Autodesk Fusion 360 part; units mm, degrees
(part 3 of 3)
sketch "Skizze23" plane through (0, 0, 15) normal (0, 0, 1) x (-1, 0, 0)
  circle A0 centre (-5.0127, -12.7944) radius 1.5
  circle A1 centre (-7.0127, 10.2056) radius 1.5
  circle A2 centre (20.7786, -30.2009) radius 1.5
  circle A3 centre (-14.804, -30.2009) radius 1.5
  circle A4 centre (12.9873, -19.7944) radius 1.5
  circle A5 centre (12.9873, 10.2056) radius 1.5
  circle A6 centre (-5.0127, 3.2056) radius 1.5
  circle A7 centre (10.9873, -12.7944) radius 1.5
  circle A8 centre (-16.9122, 11.6198) radius 1.5
  circle A9 centre (10.9873, -60.7944) radius 1.5
  circle A10 centre (-5.0127, -60.7944) radius 1.5
  circle A11 centre (-7.0127, -19.7944) radius 1.5
  circle A12 centre (22.8868, 11.6198) radius 1.5
  circle A13 centre (10.9873, 3.2056) radius 1.5
  circle A14 centre (12.9873, -49.2944) radius 1
  arc A15 (10.4462, -52.3625) -> (9.4415, -47.3835) centre (3.5497, -51.1632) ccw
  line L0 (10.4462, -52.3625) -> (9.904, -55.4797)
  arc A16 (5.9632, -58.7944) -> (9.904, -55.4797) centre (5.9632, -54.7944) ccw
  line L1 (5.9632, -58.7944) -> (0.0113, -58.7944)
  arc A17 (-3.9295, -55.4797) -> (0.0113, -58.7944) centre (0.0113, -54.7944) ccw
  line L2 (-3.9295, -55.4797) -> (-4.4716, -52.3625)
  arc A18 (-3.467, -47.3835) -> (-4.4716, -52.3625) centre (2.4249, -51.1632) ccw
  line L3 (-3.467, -47.3835) -> (1.9547, -38.932)
  arc A19 (2.7964, -38.4719) -> (1.9547, -38.932) centre (2.7964, -39.4719) ccw
  line L4 (2.7964, -38.4719) -> (3.1781, -38.4719)
  arc A20 (4.0198, -38.932) -> (3.1781, -38.4719) centre (3.1781, -39.4719) ccw
  line L5 (4.0198, -38.932) -> (9.4415, -47.3835)
  arc A21 (-4.7211, -31.3597) -> (-5.0127, -32.7585) centre (-1.5127, -32.7585) ccw
  arc A22 (-4.7211, -31.3597) -> (-4.5127, -30.3606) centre (-7.0127, -30.3606) ccw
  line L6 (-4.5127, -30.3606) -> (-4.5127, -28.821)
  arc A23 (-2.6684, -28.2852) -> (-4.5127, -28.821) centre (-3.5127, -28.821) ccw
  line L7 (-2.6684, -28.2852) -> (-0.2775, -32.0531)
  arc A24 (0.0338, -33.1247) -> (-0.2775, -32.0531) centre (-1.9662, -33.1247) ccw
  line L8 (0.0338, -33.1247) -> (0.0338, -35.784)
  arc A25 (-0.2829, -36.8639) -> (0.0338, -35.784) centre (-1.9662, -35.784) ccw
  line L9 (-0.2829, -36.8639) -> (-3.171, -41.3661)
  arc A26 (-5.0127, -40.8261) -> (-3.171, -41.3661) centre (-4.0127, -40.8261) ccw
  line L10 (-5.0127, -40.8261) -> (-5.0127, -32.7585)
  arc A27 (3.1526, -30.4719) -> (3.997, -30.0077) centre (3.1526, -29.4719) ccw
  line L11 (3.1526, -30.4719) -> (2.8219, -30.4719)
  arc A28 (1.9776, -30.0077) -> (2.8219, -30.4719) centre (2.8219, -29.4719) ccw
  line L12 (1.9776, -30.0077) -> (-0.6732, -25.8302)
  arc A29 (0.1711, -24.2944) -> (-0.6732, -25.8302) centre (0.1711, -25.2944) ccw
  line L13 (0.1711, -24.2944) -> (5.8034, -24.2944)
  arc A30 (6.6478, -25.8302) -> (5.8034, -24.2944) centre (5.8034, -25.2944) ccw
  line L14 (6.6478, -25.8302) -> (3.997, -30.0077)
  line L15 (7.9873, 8.7056) -> (-2.0127, 8.7056)
  arc A31 (-2.0127, 11.7056) -> (-2.0127, 8.7056) centre (-2.0127, 10.2056) ccw
  line L16 (-2.0127, 11.7056) -> (7.9873, 11.7056)
  arc A32 (7.9873, 8.7056) -> (7.9873, 11.7056) centre (7.9873, 10.2056) ccw
  line L17 (7.9873, -21.2944) -> (-2.0127, -21.2944)
  arc A33 (-2.0127, -18.2944) -> (-2.0127, -21.2944) centre (-2.0127, -19.7944) ccw
  line L18 (-2.0127, -18.2944) -> (7.9873, -18.2944)
  arc A34 (7.9873, -21.2944) -> (7.9873, -18.2944) centre (7.9873, -19.7944) ccw
  circle A35 centre (-7.0127, -49.2944) radius 1
  line L19 (9.4873, -1.2944) -> (9.4873, -8.2944)
  arc A36 (6.4873, -11.2944) -> (9.4873, -8.2944) centre (6.4873, -8.2944) ccw
  line L20 (6.4873, -11.2944) -> (-0.5127, -11.2944)
  arc A37 (-3.5127, -8.2944) -> (-0.5127, -11.2944) centre (-0.5127, -8.2944) ccw
  line L21 (-3.5127, -8.2944) -> (-3.5127, -1.2944)
  arc A38 (-0.5127, 1.7056) -> (-3.5127, -1.2944) centre (-0.5127, -1.2944) ccw
  line L22 (-0.5127, 1.7056) -> (6.4873, 1.7056)
  arc A39 (9.4873, -1.2944) -> (6.4873, 1.7056) centre (6.4873, -1.2944) ccw
  arc A40 (10.4873, -28.821) -> (8.6429, -28.2852) centre (9.4873, -28.821) ccw
  line L23 (10.4873, -28.821) -> (10.4873, -30.3606)
  arc A41 (10.4873, -30.3606) -> (10.6956, -31.3597) centre (12.9873, -30.3606) ccw
  arc A42 (10.9873, -32.7585) -> (10.6956, -31.3597) centre (7.4873, -32.7585) ccw
  line L24 (10.9873, -32.7585) -> (10.9873, -40.8261)
  arc A43 (9.1456, -41.3661) -> (10.9873, -40.8261) centre (9.9873, -40.8261) ccw
  line L25 (9.1456, -41.3661) -> (6.2574, -36.8639)
  arc A44 (5.9408, -35.784) -> (6.2574, -36.8639) centre (7.9408, -35.784) ccw
  line L26 (5.9408, -35.784) -> (5.9408, -33.1247)
  arc A45 (6.2521, -32.0531) -> (5.9408, -33.1247) centre (7.9408, -33.1247) ccw
  line L27 (6.2521, -32.0531) -> (8.6429, -28.2852)
  circle A46 centre (-7.0127, -29.2944) radius 1
  circle A47 centre (12.9873, -29.2944) radius 1
  arc A48 (14.4873, -45.5527) -> (15.1539, -48.0472) centre (19.4873, -45.5527) ccw
  line L28 (14.4873, -45.5527) -> (14.4873, -33.6896)
  arc A49 (17.1075, -32.6921) -> (14.4873, -33.6896) centre (15.9873, -33.6896) ccw
  line L29 (17.1075, -32.6921) -> (17.4938, -33.1258)
  arc A50 (17.4938, -33.1258) -> (24.5102, -27.8727) centre (20.7786, -30.2009) ccw
  line L30 (24.5102, -27.8727) -> (18.3167, -17.946)
  arc A51 (16.8008, -12.6526) -> (18.3167, -17.946) centre (26.8008, -12.6526) ccw
  line L31 (16.8008, -12.6526) -> (16.8008, 1.4922)
  arc A52 (20.6559, 6.3594) -> (16.8008, 1.4922) centre (21.8008, 1.4922) ccw
  line L32 (20.6559, 6.3594) -> (23.9423, 7.1324)
  arc A53 (23.9423, 7.1324) -> (22.6436, 16.2233) centre (22.8868, 11.6198) ccw
  line L33 (22.6436, 16.2233) -> (5.6243, 15.3244)
  arc A54 (0.3502, 15.3244) -> (5.6243, 15.3244) centre (2.9873, 65.2548) ccw
  line L34 (0.3502, 15.3244) -> (-16.6691, 16.2233)
  arc A55 (-16.6691, 16.2233) -> (-17.9678, 7.1324) centre (-16.9122, 11.6198) ccw
  line L35 (-17.9678, 7.1324) -> (-14.6814, 6.3594)
  arc A56 (-10.8263, 1.4922) -> (-14.6814, 6.3594) centre (-15.8263, 1.4922) ccw
  line L36 (-10.8263, 1.4922) -> (-10.8263, -12.6526)
  arc A57 (-12.3422, -17.946) -> (-10.8263, -12.6526) centre (-20.8263, -12.6526) ccw
  line L37 (-12.3422, -17.946) -> (-18.5356, -27.8727)
  arc A58 (-18.5356, -27.8727) -> (-11.5192, -33.1258) centre (-14.804, -30.2009) ccw
  line L38 (-11.5192, -33.1258) -> (-11.133, -32.6921)
  arc A59 (-8.5127, -33.6896) -> (-11.133, -32.6921) centre (-10.0127, -33.6896) ccw
  line L39 (-8.5127, -33.6896) -> (-8.5127, -45.5527)
  arc A60 (-9.1794, -48.0472) -> (-8.5127, -45.5527) centre (-13.5127, -45.5527) ccw
  arc A61 (-9.1794, -48.0472) -> (-8.9906, -50.8235) centre (-7.0127, -49.2944) ccw
  arc A62 (-8.0346, -52.946) -> (-8.9906, -50.8235) centre (-12.9463, -53.8816) ccw
  line L40 (-8.0346, -52.946) -> (-7.5111, -55.6946)
  arc A63 (-8.0639, -59.0797) -> (-7.5111, -55.6946) centre (-12.4228, -56.6301) ccw
  arc A64 (-8.0639, -59.0797) -> (-3.0273, -63.6767) centre (-5.0127, -60.7944) ccw
  arc A65 (-0.1909, -62.7944) -> (-3.0273, -63.6767) centre (-0.1909, -67.7944) ccw
  line L41 (-0.1909, -62.7944) -> (6.1654, -62.7944)
  arc A66 (9.0018, -63.6767) -> (6.1654, -62.7944) centre (6.1654, -67.7944) ccw
  arc A67 (9.0018, -63.6767) -> (14.0385, -59.0797) centre (10.9873, -60.7944) ccw
  arc A68 (13.4856, -55.6946) -> (14.0385, -59.0797) centre (18.3973, -56.6301) ccw
  line L42 (13.4856, -55.6946) -> (14.0092, -52.946)
  arc A69 (14.9651, -50.8235) -> (14.0092, -52.946) centre (18.9209, -53.8816) ccw
  arc A70 (14.9651, -50.8235) -> (15.1539, -48.0472) centre (12.9873, -49.2944) ccw
sketch "Skizze24" plane through (0, 0, 9) normal (0, 0, 1) x (-1, 0, 0)
  arc A0 (14.9683, -29.0197) -> (16.1868, -31.658) centre (19.9209, -28.333) ccw
  line L0 (16.1868, -31.658) -> (17.4938, -33.1258)
  arc A1 (17.4938, -33.1258) -> (24.5102, -27.8727) centre (20.7786, -30.2009) ccw
  line L1 (24.5102, -27.8727) -> (18.3167, -17.946)
  arc A2 (16.8008, -12.6526) -> (18.3167, -17.946) centre (26.8008, -12.6526) ccw
  line L2 (16.8008, -12.6526) -> (16.8008, 1.4922)
  arc A3 (18.2009, 4.9622) -> (16.8008, 1.4922) centre (21.8008, 1.4922) ccw
  arc A4 (19.0475, 5.6658) -> (18.2009, 4.9622) centre (28.2059, -6.2137) ccw
  arc A5 (20.6559, 6.3594) -> (19.0475, 5.6658) centre (21.8008, 1.4922) ccw
  line L3 (20.6559, 6.3594) -> (23.9423, 7.1324)
  arc A6 (23.9423, 7.1324) -> (22.935, 16.2294) centre (22.8868, 11.6198) ccw
  arc A7 (17.9873, 21.2292) -> (22.935, 16.2294) centre (22.9873, 21.2292) ccw
  line L4 (17.9873, 21.2292) -> (17.9873, 30.6994)
  arc A8 (18.5755, 33.0523) -> (17.9873, 30.6994) centre (22.9873, 30.6994) ccw
  arc A9 (18.5755, 33.0523) -> (13.2319, 37.3758) centre (15.4873, 34.6994) ccw
  arc A10 (10.01, 36.1994) -> (13.2319, 37.3758) centre (10.01, 41.1994) ccw
  line L5 (10.01, 36.1994) -> (-4.0355, 36.1994)
  arc A11 (-7.2574, 37.3758) -> (-4.0355, 36.1994) centre (-4.0355, 41.1994) ccw
  arc A12 (-7.2574, 37.3758) -> (-12.601, 33.0523) centre (-9.5127, 34.6994) ccw
  arc A13 (-12.0127, 30.6994) -> (-12.601, 33.0523) centre (-17.0127, 30.6994) ccw
  line L6 (-12.0127, 30.6994) -> (-12.0127, 21.2292)
  arc A14 (-16.9604, 16.2294) -> (-12.0127, 21.2292) centre (-17.0127, 21.2292) ccw
  arc A15 (-16.9604, 16.2294) -> (-17.9678, 7.1324) centre (-16.9122, 11.6198) ccw
  line L7 (-17.9678, 7.1324) -> (-14.6814, 6.3594)
  arc A16 (-13.0729, 5.6658) -> (-14.6814, 6.3594) centre (-15.8263, 1.4922) ccw
  arc A17 (-12.2264, 4.9622) -> (-13.0729, 5.6658) centre (-22.2314, -6.2137) ccw
  arc A18 (-10.8263, 1.4922) -> (-12.2264, 4.9622) centre (-15.8263, 1.4922) ccw
  line L8 (-10.8263, 1.4922) -> (-10.8263, -12.6526)
  arc A19 (-12.3422, -17.946) -> (-10.8263, -12.6526) centre (-20.8263, -12.6526) ccw
  line L9 (-12.3422, -17.946) -> (-18.5356, -27.8727)
  arc A20 (-18.5356, -27.8727) -> (-11.5192, -33.1258) centre (-14.804, -30.2009) ccw
  line L10 (-11.5192, -33.1258) -> (-10.2122, -31.658)
  arc A21 (-10.2122, -31.658) -> (-8.9938, -29.0197) centre (-13.9464, -28.333) ccw
  arc A22 (-7.3907, -27.3304) -> (-8.9938, -29.0197) centre (-7.0127, -29.2944) ccw
  arc A23 (-7.3907, -27.3304) -> (-5.2804, -26.3785) centre (-8.3356, -22.4205) ccw
  arc A24 (0.8301, -24.2944) -> (-5.2804, -26.3785) centre (0.8301, -34.2944) ccw
  line L11 (0.8301, -24.2944) -> (5.1444, -24.2944)
  arc A25 (11.2549, -26.3785) -> (5.1444, -24.2944) centre (5.1444, -34.2944) ccw
  arc A26 (11.2549, -26.3785) -> (13.3652, -27.3304) centre (14.3102, -22.4205) ccw
  arc A27 (14.9683, -29.0197) -> (13.3652, -27.3304) centre (12.9873, -29.2944) ccw
  line L12 (5.4873, -11.2944) -> (0.4873, -11.2944)
  arc A28 (-2.5127, -8.2944) -> (0.4873, -11.2944) centre (0.4873, -8.2944) ccw
  line L13 (-2.5127, -8.2944) -> (-2.5127, -1.2944)
  arc A29 (0.4873, 1.7056) -> (-2.5127, -1.2944) centre (0.4873, -1.2944) ccw
  line L14 (0.4873, 1.7056) -> (5.4873, 1.7056)
  arc A30 (8.4873, -1.2944) -> (5.4873, 1.7056) centre (5.4873, -1.2944) ccw
  line L15 (8.4873, -1.2944) -> (8.4873, -8.2944)
  arc A31 (5.4873, -11.2944) -> (8.4873, -8.2944) centre (5.4873, -8.2944) ccw
  line L16 (-6.0909, 17.5143) -> (1.8282, 23.1457)
  arc A32 (4.1463, 23.1457) -> (1.8282, 23.1457) centre (2.9873, 21.5158) ccw
  line L17 (4.1463, 23.1457) -> (12.0654, 17.5143)
  arc A33 (11.4859, 15.6994) -> (12.0654, 17.5143) centre (11.4859, 16.6994) ccw
  line L18 (11.4859, 15.6994) -> (-5.5113, 15.6994)
  arc A34 (-6.0909, 17.5143) -> (-5.5113, 15.6994) centre (-5.5113, 16.6994) ccw
  arc A35 (-2.0127, -18.2944) -> (-2.0127, -21.2944) centre (-2.0127, -19.7944) ccw
  line L19 (-2.0127, -18.2944) -> (7.9873, -18.2944)
  arc A36 (7.9873, -21.2944) -> (7.9873, -18.2944) centre (7.9873, -19.7944) ccw
  line L20 (7.9873, -21.2944) -> (-2.0127, -21.2944)
  line L21 (-7.0127, 22.4781) -> (-7.0127, 29.1428)
  arc A37 (-5.4332, 29.9578) -> (-7.0127, 29.1428) centre (-6.0127, 29.1428) ccw
  line L22 (-5.4332, 29.9578) -> (-0.7471, 26.6254)
  arc A38 (-0.7471, 24.9955) -> (-0.7471, 26.6254) centre (-1.3266, 25.8105) ccw
  line L23 (-0.7471, 24.9955) -> (-5.4332, 21.6632)
  arc A39 (-7.0127, 22.4781) -> (-5.4332, 21.6632) centre (-6.0127, 22.4781) ccw
  arc A40 (-0.9801, 32.6994) -> (-1.5596, 30.8844) centre (-0.9801, 31.6994) ccw
  line L24 (-0.9801, 32.6994) -> (6.9546, 32.6994)
  arc A41 (7.5342, 30.8844) -> (6.9546, 32.6994) centre (6.9546, 31.6994) ccw
  line L25 (7.5342, 30.8844) -> (4.1463, 28.4753)
  arc A42 (1.8282, 28.4753) -> (4.1463, 28.4753) centre (2.9873, 30.1052) ccw
  line L26 (1.8282, 28.4753) -> (-1.5596, 30.8844)
  line L27 (7.9873, 8.7056) -> (-2.0127, 8.7056)
  arc A43 (-2.0127, 11.7056) -> (-2.0127, 8.7056) centre (-2.0127, 10.2056) ccw
  line L28 (-2.0127, 11.7056) -> (7.9873, 11.7056)
  arc A44 (7.9873, 8.7056) -> (7.9873, 11.7056) centre (7.9873, 10.2056) ccw
  arc A45 (6.7216, 26.6254) -> (6.7216, 24.9955) centre (7.3012, 25.8105) ccw
  line L29 (6.7216, 26.6254) -> (11.4077, 29.9578)
  arc A46 (12.9873, 29.1428) -> (11.4077, 29.9578) centre (11.9873, 29.1428) ccw
  line L30 (12.9873, 29.1428) -> (12.9873, 22.4781)
  arc A47 (11.4077, 21.6632) -> (12.9873, 22.4781) centre (11.9873, 22.4781) ccw
  line L31 (11.4077, 21.6632) -> (6.7216, 24.9955)
  circle A48 centre (10.9873, 3.2056) radius 3
  circle A49 centre (-14.804, -30.2009) radius 1.5
  circle A50 centre (-16.9122, 11.6198) radius 1.5
  circle A51 centre (15.4873, 34.6994) radius 1.5
  circle A52 centre (22.8868, 11.6198) radius 1.5
  circle A53 centre (-7.0127, -19.7944) radius 1.5
  circle A54 centre (-5.0127, 3.2056) radius 3
  circle A55 centre (10.9873, -12.7944) radius 3
  circle A56 centre (20.7786, -30.2009) radius 1.5
  circle A57 centre (-7.0127, 10.2056) radius 1.5
  circle A58 centre (-9.5127, 34.6994) radius 1.5
  circle A59 centre (12.9873, 10.2056) radius 1.5
  circle A60 centre (12.9873, -19.7944) radius 1.5
  circle A61 centre (-5.0127, -12.7944) radius 3
sketch "Skizze25" plane through (0, 0, 12) normal (0, 0, 1) x (-1, 0, 0)
  circle A0 centre (-7.0127, 10.2056) radius 1.5
  circle A1 centre (-16.9122, 11.6198) radius 1.5
  circle A2 centre (-77.0127, 20.2056) radius 2.5
  line L0 (-79.9827, 16.6656) -> (-81.1827, 15.7656)
  arc A3 (-82.4427, 17.4456) -> (-81.1827, 15.7656) centre (-81.8127, 16.6056) ccw
  line L1 (-82.4427, 17.4456) -> (-81.2427, 18.3456)
  arc A4 (-79.9827, 16.6656) -> (-81.2427, 18.3456) centre (-80.6127, 17.5056) ccw
  line L2 (-71.5827, 22.9656) -> (-72.7827, 22.0656)
  arc A5 (-74.0427, 23.7456) -> (-72.7827, 22.0656) centre (-73.4127, 22.9056) ccw
  line L3 (-74.0427, 23.7456) -> (-72.8427, 24.6456)
  arc A6 (-71.5827, 22.9656) -> (-72.8427, 24.6456) centre (-72.2127, 23.8056) ccw
  line L4 (-73.4727, 17.2356) -> (-72.5727, 16.0356)
  arc A7 (-74.2527, 14.7756) -> (-72.5727, 16.0356) centre (-73.4127, 15.4056) ccw
  line L5 (-74.2527, 14.7756) -> (-75.1527, 15.9756)
  arc A8 (-73.4727, 17.2356) -> (-75.1527, 15.9756) centre (-74.3127, 16.6056) ccw
  arc A9 (-82.5459, 22.526) -> (-82.9846, 19.6249) centre (-77.0127, 20.2056) ccw
  arc A10 (-84.5885, 18.7346) -> (-82.9846, 19.6249) centre (-83.9799, 19.5281) ccw
  line L6 (-84.5885, 18.7346) -> (-87.4261, 20.9112)
  arc A11 (-87.1568, 22.6453) -> (-87.4261, 20.9112) centre (-86.8175, 21.7046) ccw
  line L7 (-87.1568, 22.6453) -> (-83.8074, 23.8534)
  arc A12 (-82.5459, 22.526) -> (-83.8074, 23.8534) centre (-83.4681, 22.9127) ccw
  arc A13 (-79.7727, 25.6356) -> (-81.4527, 24.3756) centre (-80.6127, 25.0056) ccw
  line L8 (-79.7727, 25.6356) -> (-78.8727, 24.4356)
  arc A14 (-80.5527, 23.1756) -> (-78.8727, 24.4356) centre (-79.7127, 23.8056) ccw
  line L9 (-80.5527, 23.1756) -> (-81.4527, 24.3756)
  line L10 (-43.481, 18.4383) -> (-60.0865, 20.8143)
  arc A15 (-70.5506, 25.6731) -> (-60.0865, 20.8143) centre (-57.2537, 40.6127) ccw
  arc A16 (-70.5506, 25.6731) -> (-72.7205, 26.2535) centre (-72.2127, 23.8056) ccw
  arc A17 (-76.1636, 26.1452) -> (-72.7205, 26.2535) centre (-74.7517, 36.045) ccw
  arc A18 (-79.4398, 27.2134) -> (-76.1636, 26.1452) centre (-74.7483, 36.0446) ccw
  arc A19 (-79.4398, 27.2134) -> (-81.3855, 27.3832) centre (-80.6127, 25.0056) ccw
  line L11 (-81.3855, 27.3832) -> (-91.4886, 24.0993)
  arc A20 (-91.4886, 24.0993) -> (-91.9997, 20.5467) centre (-90.8703, 22.1973) ccw
  line L12 (-91.9997, 20.5467) -> (-83.2245, 14.5424)
  arc A21 (-83.2245, 14.5424) -> (-81.3049, 14.1577) centre (-81.8127, 16.6056) ccw
  arc A22 (-77.8619, 14.266) -> (-81.3049, 14.1577) centre (-79.2738, 4.3662) ccw
  arc A23 (-74.5856, 13.1978) -> (-77.8619, 14.266) centre (-79.2772, 4.3667) ccw
  arc A24 (-74.5856, 13.1978) -> (-72.34, 13.1475) centre (-73.4127, 15.4056) ccw
  arc A25 (-60.934, 14.8819) -> (-72.34, 13.1475) centre (-63.758, -4.9177) ccw
  line L13 (-60.934, 14.8819) -> (-39.9015, 11.8821)
  arc A26 (-31.1237, 10.2271) -> (-39.9015, 11.8821) centre (-54.0217, -87.116) ccw
  line L14 (-31.1237, 10.2271) -> (-14.161, 6.237)
  arc A27 (-14.161, 6.237) -> (-9.5815, 5.7056) centre (-9.5815, 25.7056) ccw
  line L15 (-9.5815, 5.7056) -> (2.9873, 5.7056)
  line L16 (2.9873, 5.7056) -> (2.9873, 8.7056)
  line L17 (2.9873, 8.7056) -> (-2.0127, 8.7056)
  arc A28 (-2.0127, 11.7056) -> (-2.0127, 8.7056) centre (-2.0127, 10.2056) ccw
  line L18 (-2.0127, 11.7056) -> (2.9873, 11.7056)
  line L19 (2.9873, 11.7056) -> (2.9873, 15.1851)
  line L20 (2.9873, 15.1851) -> (-25.7008, 16.7003)
  arc A29 (-43.481, 18.4383) -> (-25.7008, 16.7003) centre (-15.1527, 216.4219) ccw
sketch "Skizze26" plane through (0, 0, 12) normal (0, 0, 1) x (-1, 0, 0)
  arc A0 (-8.6409, -28.1329) -> (-8.4851, -27.9011) centre (-12.7113, -25.2291) ccw
  line L0 (-8.4851, -27.9011) -> (-7.6767, -26.6224)
  arc A1 (-3.4505, -24.2944) -> (-7.6767, -26.6224) centre (-3.4505, -29.2944) ccw
  line L1 (-3.4505, -24.2944) -> (2.9873, -24.2944)
  line L2 (2.9873, -24.2944) -> (2.9873, -21.2944)
  line L3 (2.9873, -21.2944) -> (-2.0127, -21.2944)
  arc A2 (-2.0127, -18.2944) -> (-2.0127, -21.2944) centre (-2.0127, -19.7944) ccw
  line L4 (-2.0127, -18.2944) -> (2.9873, -18.2944)
  line L5 (2.9873, -18.2944) -> (2.9873, -15.2944)
  line L6 (2.9873, -15.2944) -> (-7.914, -15.2944)
  arc A3 (-7.914, -15.2944) -> (-12.1561, -17.6477) centre (-7.914, -20.2944) ccw
  line L7 (-12.1561, -17.6477) -> (-24.9738, -38.1918)
  arc A4 (-29.7754, -45.2053) -> (-24.9738, -38.1918) centre (-109.8151, 14.7418) ccw
  line L8 (-29.7754, -45.2053) -> (-46.6298, -67.7088)
  arc A5 (-56.5231, -74.7617) -> (-46.6298, -67.7088) centre (-62.6377, -55.7193) ccw
  arc A6 (-56.5231, -74.7617) -> (-58.4629, -76.7028) centre (-55.6059, -77.6181) ccw
  arc A7 (-62.3739, -81.9285) -> (-58.4629, -76.7028) centre (-67.9861, -73.6518) ccw
  arc A8 (-62.3739, -81.9285) -> (-63.6615, -83.9975) centre (-60.6902, -84.4115) ccw
  line L9 (-63.6615, -83.9975) -> (-65.1229, -94.488)
  arc A9 (-65.1229, -94.488) -> (-62.3195, -96.587) centre (-63.142, -94.7639) ccw
  line L10 (-62.3195, -96.587) -> (-52.663, -92.2303)
  arc A10 (-52.663, -92.2303) -> (-51.0398, -90.411) centre (-53.8968, -89.4957) ccw
  arc A11 (-47.1289, -85.1853) -> (-51.0398, -90.411) centre (-41.5166, -93.4619) ccw
  arc A12 (-47.1289, -85.1853) -> (-45.8135, -82.7784) centre (-48.8125, -82.7023) ccw
  arc A13 (-41.832, -71.3016) -> (-45.8135, -82.7784) centre (-25.8199, -83.2854) ccw
  line L11 (-41.832, -71.3016) -> (-24.9852, -48.7917)
  arc A14 (-19.6077, -42.2094) -> (-24.9852, -48.7917) centre (55.0754, -108.7108) ccw
  line L12 (-19.6077, -42.2094) -> (-15.1756, -37.232)
  arc A15 (-15.1756, -37.232) -> (-10.2553, -30.7009) centre (-52.5171, -3.9813) ccw
  line L13 (-10.2553, -30.7009) -> (-8.9028, -28.5618)
  arc A16 (-8.9028, -28.5618) -> (-8.7602, -28.3217) centre (-13.129, -25.8898) ccw
  arc A17 (-8.6409, -28.1329) -> (-8.7602, -28.3217) centre (-7.0127, -29.2944) ccw
  circle A18 centre (-14.804, -30.2009) radius 1.5
  circle A19 centre (-7.0127, -19.7944) radius 1.5
  arc A20 (-59.0559, -85.2371) -> (-59.355, -83.1585) centre (-59.2055, -84.1978) ccw
  line L14 (-59.0559, -85.2371) -> (-60.5406, -85.4508)
  arc A21 (-60.8397, -83.3722) -> (-60.5406, -85.4508) centre (-60.6902, -84.4115) ccw
  line L15 (-60.8397, -83.3722) -> (-59.355, -83.1585)
  arc A22 (-59.4121, -87.3355) -> (-61.1788, -87.8235) centre (-60.1889, -87.9652) ccw
  arc A23 (-59.4121, -87.3355) -> (-57.0641, -89.0932) centre (-54.7514, -83.5569) ccw
  arc A24 (-57.0349, -90.9259) -> (-57.0641, -89.0932) centre (-57.4496, -90.016) ccw
  line L16 (-57.0349, -90.9259) -> (-60.2795, -92.4046)
  arc A25 (-61.6842, -91.3529) -> (-60.2795, -92.4046) centre (-60.6943, -91.4947) ccw
  line L17 (-61.6842, -91.3529) -> (-61.1788, -87.8235)
  arc A26 (-54.5666, -77.4685) -> (-56.6452, -77.7676) centre (-55.6059, -77.6181) ccw
  line L18 (-54.5666, -77.4685) -> (-54.353, -78.9532)
  arc A27 (-56.4316, -79.2523) -> (-54.353, -78.9532) centre (-55.3923, -79.1028) ccw
  line L19 (-56.4316, -79.2523) -> (-56.6452, -77.7676)
  circle A28 centre (-54.7514, -83.5569) radius 2.5
  arc A29 (-53.0711, -87.8615) -> (-55.1497, -88.1606) centre (-54.1104, -88.011) ccw
  line L20 (-53.0711, -87.8615) -> (-52.8575, -89.3462)
  arc A30 (-54.9361, -89.6453) -> (-52.8575, -89.3462) centre (-53.8968, -89.4957) ccw
  line L21 (-54.9361, -89.6453) -> (-55.1497, -88.1606)
  line L22 (-50.4468, -81.8767) -> (-48.9621, -81.663)
  arc A31 (-48.663, -83.7416) -> (-48.9621, -81.663) centre (-48.8125, -82.7023) ccw
  line L23 (-48.663, -83.7416) -> (-50.1477, -83.9553)
  arc A32 (-50.4468, -81.8767) -> (-50.1477, -83.9553) centre (-50.2972, -82.916) ccw
component "Component" placed x (-1, 0, 0) y (0, 1, 0) z (0, 0, -1) at (-2.9873, -0.2056, 9)
component "Component'" placed x (-1, 0, 0) y (0, 1, 0) z (0, 0, -1) at (37.0127, -0.2056, 38)
component "Component''" placed x (0.6, 0.8, 0) y (0.8, -0.6, 0) z (0, 0, -1) at (-27.0049, 44.8559, 12)
component "Component'''" placed x (-0.6, 0.8, 0) y (-0.8, -0.6, 0) z (0, 0, 1) at (0.628, 28.3545, 9)
component "Component''''" placed x (-0.989831, -0.142249, 0) y (0.142249, -0.989831, 0) z (0, 0, 1) at (-29.3694, -9.1279, 9)
component "Component'''''" placed x (-1, 0, 0) y (0, 1, 0) z (0, 0, -1) at (-2.9873, -0.2056, 15)
component "Component''''''" placed x (0.989831, -0.142249, 0) y (-0.142249, -0.989831, 0) z (0, 0, -1) at (9.9638, -24.1274, 12)
